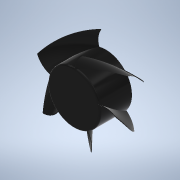
# Autodesk Inventor part: fan blade
Saved by Autodesk Inventor 2020 (Build 240168000, 168)
## iProperties
Category: Electrical
Company: Autodesk Inc.
Part Number: fan blade
Document SubType Name: Modeling
Created: 2012-11-26
Designer: Autodesk Inc.
Density: 1 g/cm^3
Material: Generic
Appearance: Glossy - Black
Control State: 0
Master: False
Checked Out: False
Shininess: 64.0
Length Units: 11272
Angle Units: 11279
Time Units: 11290
Mass Units: 11286
Length Display Precision: 3
Angle Display Precision: 2
Compacted: True
Density: 0.0
Volumn: 0.0
Area: 0.0
PropertySet Name: Model Information
Author: Autodesk Inc.
Autodesk Inventor part; units mm, degrees
ref_plane "YZ Plane" through (0, 0, 0) normal (1, 0, 0) x (0, 1, 0)
ref_plane "XZ Plane" through (0, 0, 0) normal (0, 1, 0) x (-1, 0, 0)
ref_plane "XY Plane" through (0, 0, 0) normal (0, 0, 1) x (1, 0, 0)
sketch "Sketch1" plane through (0, 0, 0) normal (0, 0, 1) x (1, 0, 0)
  circle A0 centre (20.327, 19.9052) radius 11.7286
  constraints: 1 centre point
extrude "Extrusion1" add sketch "Sketch1" along normal blind 14.3002
fillet "Fillet1" radius 0.7937 1 edges at (8.5984, 19.9052, 14.3002)
sketch "Sketch2" plane through (20.327, 19.9052, 14.3002) normal (0, 0, 1) x (1, 0, 0)
  circle A0 centre (0, 0) radius 10.9348 projected
  arc A1 (3.8809, 18.2612) -> (0.7628, 10.9082) centre (9.3054, 11.6232) ccw
  arc A2 (3.4872, 18.3448) -> (0.4428, 10.9259) centre (9.3054, 11.6232) ccw
  line L0 (3.4872, 18.3448) -> (3.8809, 18.2612)
  line L1 (0, 0) -> (0, 10.9348)
  line L2 (0, 0) -> (3.8809, 18.2612)
  line L3 (0, 0) -> (0.7628, 10.9082)
  circle A3 centre (0, 0) radius 18.669
  dimension "d7" = 37.338
  dimension "d3" = 0.3175
  dimension "d4" = 11.998
  dimension "d5" = 4
  dimension "d6" = 8.89
  constraints: 8 end point, 7 point on circle, 2 centre point, 1 coincident, 1 perpendicular, 1 vertical, 3 other
  measures "d3" radial gap between concentric circles of A1 A2
  measures "d4" angle of L1 L2
  measures "d5" angle of L1 L3
  measures "d6" radius of A2
coil "Coil1" sketch "Sketch2" operation add axis through (20.327, 19.9052, 0) along (0, 0, -1) pitch 95.3347 turns 0.15 hand right contours A0 A2 A3 A1 | A3 A2 L0
pattern_circular "Circular Pattern1" count 5 over 360 about axis through (20.327, 19.9052, 0) along (0, 0, 1) of "Coil1"
body "Solid1"
